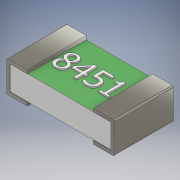
# Autodesk Inventor part: 21-1001
Saved by Autodesk Inventor 2018 (Build 220112000, 112)
## iProperties
Created: 2019-09-21
Part Number: 21-1001
Material: Copper
Document SubType Name: Modeling
Designer: Bradley
Density: 8.94 g/cm^3
Appearance: Smooth - White
Author: Bradley
Autodesk Inventor part; units mm, degrees
ref_plane "YZ Plane" through (0, 0, 0) normal (1, 0, 0) x (0, 1, 0)
ref_plane "XZ Plane" through (0, 0, 0) normal (0, 1, 0) x (-1, 0, 0)
ref_plane "XY Plane" through (0, 0, 0) normal (0, 0, 1) x (1, 0, 0)
sketch "Sketch1" plane through (0, 0, 0) normal (0, 1, 0) x (-1, 0, 0)
  line L0 (0.725, 0.175) -> (-0.725, 0.175)
  line L1 (-0.725, 0.175) -> (-0.725, -0.175)
  line L2 (-0.725, -0.175) -> (0.725, -0.175)
  line L3 (0.725, -0.175) -> (0.725, 0.175)
  line L4 (0.475, 0.175) -> (0.475, 0.225)
  line L5 (0.475, 0.225) -> (0.775, 0.225)
  line L6 (0.775, 0.225) -> (0.775, -0.225)
  line L7 (0.775, -0.225) -> (0.475, -0.225)
  line L8 (0.475, -0.225) -> (0.475, -0.175)
  line L9 (-0.475, 0.175) -> (-0.475, 0.225)
  line L10 (-0.475, 0.225) -> (-0.775, 0.225)
  line L11 (-0.775, 0.225) -> (-0.775, -0.225)
  line L12 (-0.775, -0.225) -> (-0.475, -0.225)
  line L13 (-0.475, -0.175) -> (-0.475, -0.225)
  line L14 (0.475, 0.175) -> (-0.475, 0.175)
  point P0 (0, 0)
  point P1 (0, 0.175)
  point P2 (0.725, 0)
  dimension "d0" = 1.55
  dimension "d1" = 0.05
  dimension "d2" = 0.05
  dimension "d3" = 0.45
  dimension "d4" = 0.3
  constraints: 30 end point, 12 point on line, 7 perpendicular, 3 collinear, 3 midpoint, 2 parallel, 1 horizontal, 1 horizontal alignment, 1 vertical, 1 vertical alignment
  measures "d0" distance between parallel lines of L11 L6
  measures "d1" distance of L7.end L8.end
  measures "d2" distance between parallel lines of L6 L3
  measures "d3" distance of L5.end L6.end
  measures "d4" distance of L6.end L7.end
extrude "Extrusion1" add sketch "Sketch1" along normal mid plane 0.85 contours L0 L4 L5 L6 L7 L8 L2 L3 | L0 L1 L2 L13 L12 L11 L10 L9
extrude "Extrusion2" add sketch "Sketch1" along normal mid plane 0.84 contours L3 L2 L1 L0
sketch "Sketch2" plane through (-0.475, -0.42, 0.175) normal (0, 0, 1) x (1, 0, 0)
  line L0 (0, 0) -> (0, 0.84) projected
  line L1 (0.95, 0) -> (0, 0) projected
  line L2 (0.95, 0) -> (0.95, 0.84) projected
  line L3 (0, 0.84) -> (0.95, 0.84) projected
  line L4 (0, 0.42) -> (0.95, 0.42) construction
  spline S0 degree 2 poles (0.1373, 0.2632) (0.115, 0.2632) (0.0782, 0.2766) (0.0654, 0.289) knots 0 0 0 1 2 2 2
  spline S1 degree 2 poles (0.0654, 0.289) (0.0527, 0.3011) (0.0396, 0.3342) (0.0396, 0.3529) knots 0 0 0 1 2 2 2
  spline S2 degree 2 poles (0.0396, 0.3529) (0.0396, 0.3772) (0.0656, 0.4181) (0.0904, 0.4302) knots 0 0 0 1 2 2 2
  line L5 (0.0904, 0.4302) -> (0.0904, 0.4314)
  spline S3 degree 2 poles (0.0904, 0.4314) (0.0683, 0.4443) (0.0469, 0.4749) (0.0469, 0.4978) knots 0 0 0 1 2 2 2
  spline S4 degree 2 poles (0.0469, 0.4978) (0.0469, 0.5316) (0.0979, 0.5768) (0.1373, 0.5768) knots 0 0 0 1 2 2 2
  spline S5 degree 2 poles (0.1373, 0.5768) (0.1782, 0.5768) (0.2275, 0.534) (0.2275, 0.5005) knots 0 0 0 1 2 2 2
  spline S6 degree 2 poles (0.2275, 0.5005) (0.2275, 0.4803) (0.2039, 0.4409) (0.1818, 0.4297) knots 0 0 0 1 2 2 2
  line L6 (0.1818, 0.4297) -> (0.1818, 0.4285)
  spline S7 degree 2 poles (0.1818, 0.4285) (0.2081, 0.4164) (0.235, 0.3813) (0.235, 0.3536) knots 0 0 0 1 2 2 2
  spline S8 degree 2 poles (0.235, 0.3536) (0.235, 0.3152) (0.1791, 0.2632) (0.1373, 0.2632) knots 0 0 0 1 2 2 2
  spline S9 degree 2 poles (0.1937, 0.3497) (0.1937, 0.3682) (0.1791, 0.3901) (0.1585, 0.4013) knots 0 0 0 1 2 2 2
  spline S10 degree 2 poles (0.1585, 0.4013) (0.1517, 0.4052) (0.1288, 0.4142) (0.1145, 0.42) knots 0 0 0 1 2 2 2
  spline S11 degree 2 poles (0.1145, 0.42) (0.0979, 0.4091) (0.0802, 0.3765) (0.0802, 0.3558) knots 0 0 0 1 2 2 2
  spline S12 degree 2 poles (0.0802, 0.3558) (0.0802, 0.3286) (0.113, 0.2931) (0.1378, 0.2931) knots 0 0 0 1 2 2 2
  spline S13 degree 2 poles (0.1378, 0.2931) (0.1631, 0.2931) (0.1937, 0.3235) (0.1937, 0.3497) knots 0 0 0 1 2 2 2
  spline S14 degree 2 poles (0.1881, 0.5) (0.1881, 0.5202) (0.1611, 0.5471) (0.1371, 0.5471) knots 0 0 0 1 2 2 2
  spline S15 degree 2 poles (0.1371, 0.5471) (0.1152, 0.5471) (0.0872, 0.5231) (0.0872, 0.5024) knots 0 0 0 1 2 2 2
  spline S16 degree 2 poles (0.0872, 0.5024) (0.0872, 0.4876) (0.1016, 0.4669) (0.1159, 0.4587) knots 0 0 0 1 2 2 2
  spline S17 degree 2 poles (0.1159, 0.4587) (0.122, 0.4553) (0.1478, 0.4433) (0.1582, 0.4399) knots 0 0 0 1 2 2 2
  spline S18 degree 2 poles (0.1582, 0.4399) (0.1757, 0.4533) (0.1881, 0.4818) (0.1881, 0.5) knots 0 0 0 1 2 2 2
  line L7 (0.4648, 0.3731) -> (0.4291, 0.3731)
  line L8 (0.4291, 0.3731) -> (0.4291, 0.27)
  line L9 (0.4291, 0.27) -> (0.3904, 0.27)
  line L10 (0.3904, 0.27) -> (0.3904, 0.3731)
  line L11 (0.3904, 0.3731) -> (0.2579, 0.3731)
  line L12 (0.2579, 0.3731) -> (0.2579, 0.4154)
  line L13 (0.2579, 0.4154) -> (0.3921, 0.57)
  line L14 (0.3921, 0.57) -> (0.4291, 0.57)
  line L15 (0.4291, 0.57) -> (0.4291, 0.4054)
  line L16 (0.4291, 0.4054) -> (0.4648, 0.4054)
  line L17 (0.4648, 0.4054) -> (0.4648, 0.3731)
  line L18 (0.3904, 0.4054) -> (0.3904, 0.5226)
  line L19 (0.3904, 0.5226) -> (0.2895, 0.4054)
  line L20 (0.2895, 0.4054) -> (0.3904, 0.4054)
  spline S19 degree 2 poles (0.6787, 0.3653) (0.6787, 0.3437) (0.6649, 0.3067) (0.6522, 0.2931) knots 0 0 0 1 2 2 2
  spline S20 degree 2 poles (0.6522, 0.2931) (0.6396, 0.2795) (0.6019, 0.2637) (0.5786, 0.2637) knots 0 0 0 1 2 2 2
  spline S21 degree 2 poles (0.5786, 0.2637) (0.5572, 0.2637) (0.5154, 0.2732) (0.5, 0.2807) knots 0 0 0 1 2 2 2
  line L21 (0.5, 0.2807) -> (0.5, 0.3232)
  line L22 (0.5, 0.3232) -> (0.503, 0.3232)
  spline S22 degree 2 poles (0.503, 0.3232) (0.5076, 0.3198) (0.5248, 0.3111) (0.5353, 0.3072) knots 0 0 0 1 2 2 2
  spline S23 degree 2 poles (0.5353, 0.3072) (0.5472, 0.3031) (0.5669, 0.2984) (0.5793, 0.2984) knots 0 0 0 1 2 2 2
  spline S24 degree 2 poles (0.5793, 0.2984) (0.5915, 0.2984) (0.6143, 0.3072) (0.6226, 0.3167) knots 0 0 0 1 2 2 2
  spline S25 degree 2 poles (0.6226, 0.3167) (0.6301, 0.3257) (0.6379, 0.3495) (0.6379, 0.3655) knots 0 0 0 1 2 2 2
  spline S26 degree 2 poles (0.6379, 0.3655) (0.6379, 0.3816) (0.6291, 0.402) (0.6209, 0.4088) knots 0 0 0 1 2 2 2
  spline S27 degree 2 poles (0.6209, 0.4088) (0.6124, 0.4164) (0.5871, 0.4227) (0.5718, 0.4227) knots 0 0 0 1 2 2 2
  spline S28 degree 2 poles (0.5718, 0.4227) (0.5552, 0.4227) (0.5224, 0.4176) (0.5124, 0.4154) knots 0 0 0 1 2 2 2
  line L23 (0.5124, 0.4154) -> (0.5124, 0.57)
  line L24 (0.5124, 0.57) -> (0.677, 0.57)
  line L25 (0.677, 0.57) -> (0.677, 0.5347)
  line L26 (0.677, 0.5347) -> (0.5511, 0.5347)
  line L27 (0.5511, 0.5347) -> (0.5511, 0.4548)
  spline S29 degree 2 poles (0.5511, 0.4548) (0.5584, 0.4557) (0.5725, 0.4565) (0.5783, 0.4565) knots 0 0 0 1 2 2 2
  spline S30 degree 2 poles (0.5783, 0.4565) (0.6014, 0.4565) (0.6333, 0.4489) (0.6479, 0.4377) knots 0 0 0 1 2 2 2
  spline S31 degree 2 poles (0.6479, 0.4377) (0.6627, 0.4266) (0.6787, 0.3925) (0.6787, 0.3653) knots 0 0 0 1 2 2 2
  line L28 (0.8919, 0.27) -> (0.7456, 0.27)
  line L29 (0.7456, 0.27) -> (0.7456, 0.3006)
  line L30 (0.7456, 0.3006) -> (0.8, 0.3006)
  line L31 (0.8, 0.3006) -> (0.8, 0.5017)
  line L32 (0.8, 0.5017) -> (0.7456, 0.5017)
  line L33 (0.7456, 0.5017) -> (0.7456, 0.5292)
  spline S32 degree 2 poles (0.7456, 0.5292) (0.7765, 0.5292) (0.8056, 0.5467) (0.8076, 0.571) knots 0 0 0 1 2 2 2
  line L34 (0.8076, 0.571) -> (0.8387, 0.571)
  line L35 (0.8387, 0.571) -> (0.8387, 0.3006)
  line L36 (0.8387, 0.3006) -> (0.8919, 0.3006)
  line L37 (0.8919, 0.3006) -> (0.8919, 0.27)
  point P0 (0.475, 0.42)
  constraints: 2 end point, 2 midpoint, 1 horizontal
extrude "Extrusion3" add sketch "Sketch2" along normal blind 0.02 contours S0 S1 S2 S3 S4 S5 S6 S7 S8 | L7 L8 L9 L10 L11 L12 L13 L14 L15 L16 L17 | S19 S20 S21 L21 L22 S22 S23 S24 S25 S26 S27 S28 L23 L24 L25 L26 L27 S29 S30 S31 | L28 L29 L30 L31 L32 L33 S32 L34 L35 L36 L37
fillet "Fillet1" radius 0.02 4 edges at (-0.775, 0, 0.225) (-0.775, 0, -0.225) (0.775, 0, 0.225) (0.775, 0, -0.225)
equation "\"d2\" = d1"
body "Solid1"
